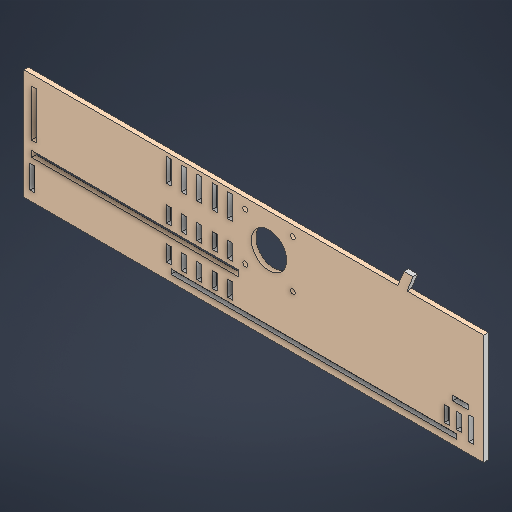
# Autodesk Inventor part: Sideboard
Saved by Autodesk Inventor 2027 (Build 310192000, 192)
## iProperties
Created: 2026-05-09
Part Number: Sideboard
Material: Generic
Document SubType Name: Modeling
Designer: alexy
Density: 1 g/cm^3
Appearance: Default
Author: alexy
Autodesk Inventor part; units mm, degrees
ref_plane "YZ Plane" through (0, 0, 0) normal (1, 0, 0) x (0, 1, 0)
ref_plane "XZ Plane" through (0, 0, 0) normal (0, 1, 0) x (-1, 0, 0)
ref_plane "XY Plane" through (0, 0, 0) normal (0, 0, 1) x (1, 0, 0)
sketch "Sketch1" plane through (0, 0, 0) normal (0, 0, 1) x (1, 0, 0)
  line L0 (0, 0) -> (300, 0)
  line L1 (300, 0) -> (300, 62)
  line L2 (300, 62) -> (0, 62)
  line L3 (0, 62) -> (0, 0)
  circle A0 centre (144.5, 55.5) radius 1.55
  circle A1 centre (144.5, 24.5) radius 1.55
  circle A2 centre (175.5, 55.5) radius 1.55
  circle A3 centre (175.5, 24.5) radius 1.55
  circle A4 centre (160, 40) radius 11.5
  line L4 (5, 19) -> (140, 19)
  line L5 (140, 19) -> (140, 15)
  line L6 (140, 15) -> (5, 15)
  line L7 (5, 15) -> (5, 19)
  line L8 (0, 62) -> (39.6145, 62)
  line L9 (8.1, 24.8) -> (5, 24.8)
  line L10 (5, 24.8) -> (5, 55.2)
  line L11 (5, 55.2) -> (8.1, 55.2)
  line L12 (8.1, 55.2) -> (8.1, 24.8)
  line L13 (8.1, 24.8) -> (5, 55.2) construction
  line L14 (5, 24.8) -> (8.1, 55.2) construction
  line L15 (0, 62) -> (50, 62)
  line L16 (0, 0) -> (0, -10)
  line L17 (0, -10) -> (300, -10)
  line L18 (300, -10) -> (300, 0)
  point P0 (6.55, 40)
  point P1 (5, 40)
  point P2 (8.1, 40)
  point P3 (5, 17)
  point P4 (140, 17)
  dimension "d1" = 3.1
  dimension "d2" = 3.1
  dimension "d3" = 3.1
  dimension "d4" = 3.1
  dimension "d5" = 31
  dimension "d7" = 23
  dimension "d8" = 15.5
  dimension "d9" = 15.5
  dimension "d10" = 62
  dimension "d11" = 31
  dimension "d13" = 40
  dimension "d54" = 300
  dimension "d55" = 3.1
  dimension "d56" = 5
  dimension "d57" = 15.2
  dimension "d59" = 135
  dimension "d93" = 15
  dimension "d106" = 20
  dimension "d107" = 5
  dimension "d201" = 4
  dimension "d202" = 10
  constraints: 38 end point, 6 midpoint, 6 parallel, 5 centre point, 5 perpendicular, 4 horizontal, 3 horizontal alignment, 2 vertical alignment, 1 vertical
  measures "d1" diameter of A0
  measures "d2" diameter of A1
  measures "d3" diameter of A2
  measures "d4" diameter of A3
  measures "d5" distance of A1.centre A3.centre
  measures "d7" diameter of A4
  measures "d8" horizontal distance of A0.centre A4.centre
  measures "d9" horizontal distance of A4.centre A3.centre
  measures "d10" distance of L0.end L1.end
  measures "d11" distance of A3.centre A2.centre
  measures "d13" distance from line of L0 A4.centre
  measures "d54" distance of L0.end L0.start
  measures "d55" distance of L10.end L11.end
  measures "d56" distance between parallel lines of L3 L10
  measures "d57" distance of point (5, 40) L10.end
  measures "d59" distance of L5.end L6.end
  measures "d93" distance between parallel lines of L0 L6
  measures "d106" horizontal distance of point (140, 17) A4.centre
  measures "d107" distance from line of L3 point (5, 17)
  measures "d201" distance of L6.end L4.start
  measures "d202" distance of L0.start L16.end
extrude "Extrusion1" add sketch "Sketch1" along normal blind 3
sketch "Sketch4" plane through (0, 0, 3) normal (0, 0, 1) x (1, 0, 0)
  line L0 (300, 62) -> (0, 62) projected
  line L1 (244, 62) -> (248, 72)
  line L2 (248, 72) -> (254, 72)
  line L3 (254, 72) -> (250, 62)
  line L4 (0, -10) -> (300, -10) projected
  point P0 (0, 0)
  dimension "d108" = 10
  dimension "d109" = 4
  dimension "d110" = 50
  dimension "d111" = 6
  constraints: 6 end point, 2 parallel, 2 point on line
  measures "d108" distance from line of L0 L1.end
  measures "d109" horizontal distance of L1.start L1.end
  measures "d110" distance of L0.start L3.end
  measures "d111" distance of L2.end L1.end
extrude "Extrusion4" add sketch "Sketch4" against normal blind 3
sketch "Sketch7" plane through (0, 0, 3) normal (0, 0, 1) x (1, 0, 0)
  line L0 (132.9, 59.6) -> (136.1, 59.6)
  line L1 (136.1, 59.6) -> (136.1, 44.4)
  line L2 (136.1, 44.4) -> (132.9, 44.4)
  line L3 (132.9, 44.4) -> (132.9, 59.6)
  line L4 (132.9, 59.6) -> (136.1, 44.4) construction
  line L5 (136.1, 59.6) -> (132.9, 44.4) construction
  line L6 (132.9, 32.1) -> (136.1, 32.1)
  line L7 (136.1, 32.1) -> (136.1, 21.9)
  line L8 (136.1, 21.9) -> (132.9, 21.9)
  line L9 (132.9, 21.9) -> (132.9, 32.1)
  line L10 (132.9, 32.1) -> (136.1, 21.9) construction
  line L11 (136.1, 32.1) -> (132.9, 21.9) construction
  line L12 (244, 62) -> (0, 62) projected
  circle A0 centre (144.5, 55.5) radius 1.55 projected
  line L13 (122.9, 59.6) -> (126.1, 59.6)
  line L14 (126.1, 59.6) -> (126.1, 44.4)
  line L15 (126.1, 44.4) -> (122.9, 44.4)
  line L16 (122.9, 44.4) -> (122.9, 59.6)
  line L17 (122.9, 59.6) -> (126.1, 44.4) construction
  line L18 (126.1, 59.6) -> (122.9, 44.4) construction
  line L19 (122.9, 32.1) -> (126.1, 32.1)
  line L20 (126.1, 32.1) -> (126.1, 21.9)
  line L21 (126.1, 21.9) -> (122.9, 21.9)
  line L22 (122.9, 21.9) -> (122.9, 32.1)
  line L23 (122.9, 32.1) -> (126.1, 21.9) construction
  line L24 (126.1, 32.1) -> (122.9, 21.9) construction
  line L25 (112.9, 59.6) -> (116.1, 59.6)
  line L26 (116.1, 59.6) -> (116.1, 44.4)
  line L27 (116.1, 44.4) -> (112.9, 44.4)
  line L28 (112.9, 44.4) -> (112.9, 59.6)
  line L29 (112.9, 59.6) -> (116.1, 44.4) construction
  line L30 (116.1, 59.6) -> (112.9, 44.4) construction
  line L31 (112.9, 32.1) -> (116.1, 32.1)
  line L32 (116.1, 32.1) -> (116.1, 21.9)
  line L33 (116.1, 21.9) -> (112.9, 21.9)
  line L34 (112.9, 21.9) -> (112.9, 32.1)
  line L35 (112.9, 32.1) -> (116.1, 21.9) construction
  line L36 (116.1, 32.1) -> (112.9, 21.9) construction
  line L37 (102.9, 59.6) -> (106.1, 59.6)
  line L38 (106.1, 59.6) -> (106.1, 44.4)
  line L39 (106.1, 44.4) -> (102.9, 44.4)
  line L40 (102.9, 44.4) -> (102.9, 59.6)
  line L41 (102.9, 59.6) -> (106.1, 44.4) construction
  line L42 (106.1, 59.6) -> (102.9, 44.4) construction
  line L43 (102.9, 32.1) -> (106.1, 32.1)
  line L44 (106.1, 32.1) -> (106.1, 21.9)
  line L45 (106.1, 21.9) -> (102.9, 21.9)
  line L46 (102.9, 21.9) -> (102.9, 32.1)
  line L47 (102.9, 32.1) -> (106.1, 21.9) construction
  line L48 (106.1, 32.1) -> (102.9, 21.9) construction
  line L49 (92.9, 59.6) -> (96.1, 59.6)
  line L50 (96.1, 59.6) -> (96.1, 44.4)
  line L51 (96.1, 44.4) -> (92.9, 44.4)
  line L52 (92.9, 44.4) -> (92.9, 59.6)
  line L53 (92.9, 59.6) -> (96.1, 44.4) construction
  line L54 (96.1, 59.6) -> (92.9, 44.4) construction
  line L55 (92.9, 32.1) -> (96.1, 32.1)
  line L56 (96.1, 32.1) -> (96.1, 21.9)
  line L57 (96.1, 21.9) -> (92.9, 21.9)
  line L58 (92.9, 21.9) -> (92.9, 32.1)
  line L59 (92.9, 32.1) -> (96.1, 21.9) construction
  line L60 (96.1, 32.1) -> (92.9, 21.9) construction
  line L61 (132.9, 10.1) -> (136.1, 10.1)
  line L62 (136.1, 10.1) -> (136.1, -0.1)
  line L63 (136.1, -0.1) -> (132.9, -0.1)
  line L64 (132.9, -0.1) -> (132.9, 10.1)
  line L65 (132.9, 10.1) -> (136.1, -0.1) construction
  line L66 (136.1, 10.1) -> (132.9, -0.1) construction
  line L67 (126.1, 10.1) -> (126.1, -0.1)
  line L68 (126.1, -0.1) -> (122.9, -0.1)
  line L69 (122.9, 10.1) -> (126.1, 10.1)
  line L70 (122.9, -0.1) -> (122.9, 10.1)
  line L71 (122.9, 10.1) -> (126.1, -0.1) construction
  line L72 (126.1, 10.1) -> (122.9, -0.1) construction
  line L73 (116.1, 10.1) -> (116.1, -0.1)
  line L74 (116.1, -0.1) -> (112.9, -0.1)
  line L75 (112.9, 10.1) -> (116.1, 10.1)
  line L76 (112.9, -0.1) -> (112.9, 10.1)
  line L77 (112.9, 10.1) -> (116.1, -0.1) construction
  line L78 (116.1, 10.1) -> (112.9, -0.1) construction
  line L79 (106.1, 10.1) -> (106.1, -0.1)
  line L80 (106.1, -0.1) -> (102.9, -0.1)
  line L81 (102.9, 10.1) -> (106.1, 10.1)
  line L82 (102.9, -0.1) -> (102.9, 10.1)
  line L83 (102.9, 10.1) -> (106.1, -0.1) construction
  line L84 (106.1, 10.1) -> (102.9, -0.1) construction
  line L85 (96.1, 10.1) -> (96.1, -0.1)
  line L86 (96.1, -0.1) -> (92.9, -0.1)
  line L87 (92.9, 10.1) -> (96.1, 10.1)
  line L88 (92.9, -0.1) -> (92.9, 10.1)
  line L89 (92.9, 10.1) -> (96.1, -0.1) construction
  line L90 (96.1, 10.1) -> (92.9, -0.1) construction
  line L91 (0, -10) -> (300, -10) projected
  point P0 (0, 0)
  point P1 (134.5, 52)
  point P2 (134.5, 27)
  point P3 (124.5, 52)
  point P4 (124.5, 27)
  point P5 (114.5, 52)
  point P6 (114.5, 27)
  point P7 (104.5, 52)
  point P8 (104.5, 27)
  point P9 (94.5, 52)
  point P10 (94.5, 27)
  point P11 (132.9, 52)
  point P12 (112.9, 52)
  point P13 (134.5, 5)
  point P14 (124.5, 5)
  point P15 (114.5, 5)
  point P16 (104.5, 5)
  point P17 (94.5, 5)
  point P18 (132.9, 5)
  point P19 (112.9, 5)
  point P20 (150, -10)
  dimension "d147" = 3.2
  dimension "d148" = 15.2
  dimension "d149" = 10.2
  dimension "d150" = 25
  dimension "d151" = 10
  dimension "d152" = 10
  dimension "d153" = 3.2
  dimension "d154" = 15.2
  dimension "d155" = 10.2
  dimension "d156" = 25
  dimension "d157" = 3.2
  dimension "d158" = 15.2
  dimension "d159" = 10.2
  dimension "d160" = 25
  dimension "d161" = 3.2
  dimension "d162" = 15.2
  dimension "d163" = 10.2
  dimension "d164" = 25
  dimension "d165" = 3.2
  dimension "d166" = 15.2
  dimension "d167" = 10.2
  dimension "d168" = 25
  dimension "d169" = 10
  dimension "d170" = 10
  dimension "d171" = 10
  dimension "d172" = 10
  dimension "d181" = 3.2
  dimension "d183" = 3.2
  dimension "d185" = 3.2
  dimension "d187" = 3.2
  dimension "d189" = 3.2
  dimension "d191" = 10
  dimension "d192" = 10
  dimension "d193" = 10
  dimension "d194" = 10
  dimension "d234" = 15
  dimension "d235" = 10.2
  constraints: 180 end point, 35 midpoint, 30 parallel, 15 horizontal, 15 perpendicular, 12 horizontal alignment, 6 vertical alignment, 5 point on line
  measures "d147" distance of L1.end L2.end
  measures "d148" distance of L2.end L0.start
  measures "d149" distance of L8.end L6.start
  measures "d150" distance of point (134.5, 27) point (134.5, 52)
  measures "d151" distance from line of L12 point (134.5, 52)
  measures "d152" horizontal distance of A0.centre point (134.5, 52)
  measures "d153" distance of L14.end L15.end
  measures "d154" distance of L15.end L13.start
  measures "d155" distance of L22.start L19.start
  measures "d156" distance of point (124.5, 27) point (124.5, 52)
  measures "d157" distance of L26.end L27.end
  measures "d158" distance of L27.end L25.start
  measures "d159" distance of L34.start L31.start
  measures "d160" distance of point (114.5, 27) point (114.5, 52)
  measures "d161" distance of L38.end L39.end
  measures "d162" distance of L39.end L37.start
  measures "d163" distance of L46.start L43.start
  measures "d164" distance of point (104.5, 27) point (104.5, 52)
  measures "d165" distance of L50.end L51.end
  measures "d166" distance of L51.end L49.start
  measures "d167" distance of L58.start L55.start
  measures "d168" distance of point (94.5, 27) point (94.5, 52)
  measures "d169" distance of point (124.5, 52) point (134.5, 52)
  measures "d170" distance of point (124.5, 52) point (114.5, 52)
  measures "d171" distance of point (104.5, 52) point (114.5, 52)
  measures "d172" distance of point (94.5, 52) point (104.5, 52)
  measures "d181" distance of L63.start L63.end
  measures "d183" distance of L67.end L70.start
  measures "d185" distance of L73.end L78.end
  measures "d187" distance of L79.end L82.start
  measures "d189" distance of L85.end L86.end
  measures "d191" distance of point (124.5, 5) point (134.5, 5)
  measures "d192" distance of point (124.5, 5) point (114.5, 5)
  measures "d193" distance of point (104.5, 5) point (114.5, 5)
  measures "d194" distance of point (94.5, 5) point (104.5, 5)
  measures "d234" vertical distance of point (150, -10) point (134.5, 5)
  measures "d235" distance of L62.start L63.start
extrude "Extrusion6" cut sketch "Sketch7" against normal blind 3 contours L0 L1 L2 L3 | L6 L7 L8 L9 | L13 L14 L15 L16 | L19 L20 L21 L22 | L25 L26 L27 L28 | L31 L32 L33 L34 | L37 L38 L39 L40 | L43 L44 L45 L46 | L49 L50 L51 L52 | L55 L56 L57 L58 | L61 L62 L63 L64 | L67 L68 L70 L69 | L73 L74 L76 L75 | L79 L80 L82 L81 | L85 L86 L88 L87
sketch "Sketch8" plane through (0, 0, 3) normal (0, 0, 1) x (1, 0, 0)
  line L0 (0, -10) -> (300, -10) projected
  line L1 (279.8, 18) -> (290, 18)
  line L2 (290, 18) -> (290, 14.8)
  line L3 (290, 14.8) -> (279.8, 14.8)
  line L4 (279.8, 14.8) -> (279.8, 18)
  line L5 (300, -10) -> (300, 62) projected
  line L6 (4, 11.2) -> (7.2, 11.2)
  line L7 (7.2, 11.2) -> (7.2, -4)
  line L8 (7.2, -4) -> (4, -4)
  line L9 (4, -4) -> (4, 11.2)
  line L10 (4, 11.2) -> (7.2, -4) construction
  line L11 (7.2, 11.2) -> (4, -4) construction
  line L12 (282.4, 10.1) -> (285.6, 10.1)
  line L13 (285.6, 10.1) -> (285.6, -0.1)
  line L14 (285.6, -0.1) -> (282.4, -0.1)
  line L15 (282.4, -0.1) -> (282.4, 10.1)
  line L16 (282.4, 10.1) -> (285.6, -0.1) construction
  line L17 (285.6, 10.1) -> (282.4, -0.1) construction
  line L18 (274.4, 10.1) -> (277.6, 10.1)
  line L19 (277.6, 10.1) -> (277.6, -0.1)
  line L20 (277.6, -0.1) -> (274.4, -0.1)
  line L21 (274.4, -0.1) -> (274.4, 10.1)
  line L22 (274.4, 10.1) -> (277.6, -0.1) construction
  line L23 (277.6, 10.1) -> (274.4, -0.1) construction
  line L24 (96.1, -2.45) -> (282.4, -2.45)
  line L25 (282.4, -2.45) -> (282.4, -5.55)
  line L26 (282.4, -5.55) -> (96.1, -5.55)
  line L27 (96.1, -5.55) -> (96.1, -2.45)
  line L28 (96.1, -2.45) -> (282.4, -5.55) construction
  line L29 (282.4, -2.45) -> (96.1, -5.55) construction
  line L30 (136.1, 10.1) -> (136.1, -0.1) projected
  line L31 (290.4, 12.2) -> (293.6, 12.2)
  line L32 (293.6, 12.2) -> (293.6, -3)
  line L33 (293.6, -3) -> (290.4, -3)
  line L34 (290.4, -3) -> (290.4, 12.2)
  line L35 (290.4, 12.2) -> (293.6, -3) construction
  line L36 (293.6, 12.2) -> (290.4, -3) construction
  point P0 (0, 0)
  point P1 (5.6, 3.6)
  point P2 (4, 3.6)
  point P3 (284, 5)
  point P4 (282.4, 5)
  point P5 (276, 5)
  point P6 (274.4, 5)
  point P7 (189.25, -4)
  point P8 (136.1, 5)
  point P9 (96.1, -0.1)
  point P10 (292, 4.6)
  dimension "d219" = 28
  dimension "d220" = 3.2
  dimension "d221" = 10.2
  dimension "d222" = 10
  dimension "d223" = 3.2
  dimension "d224" = 15.2
  dimension "d225" = 4
  dimension "d226" = 6
  dimension "d227" = 3.2
  dimension "d229" = 3.2
  dimension "d232" = 8
  dimension "d233" = 15
  dimension "d236" = 3.1
  dimension "d237" = 9
  dimension "d238" = 10.2
  dimension "d240" = 3.2
  dimension "d241" = 15.2
  dimension "d242" = 7
  dimension "d243" = 16
  dimension "d244" = 8
  constraints: 68 end point, 14 midpoint, 12 parallel, 6 horizontal, 6 perpendicular, 3 horizontal alignment, 2 vertical alignment
  measures "d219" distance between parallel lines of L0 L1
  measures "d220" distance of L3.end L1.start
  measures "d221" distance of L2.end L3.end
  measures "d222" distance between parallel lines of L5 L2
  measures "d223" distance of L7.end L8.end
  measures "d224" distance of L6.end L7.end
  measures "d225" horizontal distance of L0.start L8.end
  measures "d226" vertical distance of L0.start L8.end
  measures "d227" distance of L16.end L15.start
  measures "d229" distance of L22.end L21.start
  measures "d232" distance of point (276, 5) point (284, 5)
  measures "d233" distance from line of L0 point (276, 5)
  measures "d236" distance of L26.end L24.start
  measures "d237" vertical distance of point (189.25, -4) point (136.1, 5)
  measures "d238" distance of L12.end L16.end
  measures "d240" distance of L32.end L33.end
  measures "d241" distance of L31.end L32.end
  measures "d242" distance between parallel lines of L0 L33
  measures "d243" horizontal distance of L0.end point (284, 5)
  measures "d244" horizontal distance of L0.end point (292, 4.6)
extrude "Extrusion7" cut sketch "Sketch8" against normal blind 3
body "Solid1"
